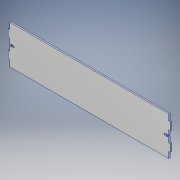
# Autodesk Inventor part: Hopper Leg Brace
Saved by Autodesk Inventor 2018 (Build 220112000, 112)
## iProperties
Created: 2013-10-29
Part Number: Hopper Leg Brace
Material: Aluminum 6061
Document SubType Name: Modeling
Designer: Gabriel Smolnycki
Mass: 474.034 g
Surface Area: 923.52 cm^2
Volume: 175.568 cm^3
Density: 2.7 g/cm^3
Appearance: Aluminum - Flat
Sending System: SolidWorks 2017
Last Author: Gabriel Smolnycki
Last Saved: 2017-09-14
Author: Gabriel Smolnycki
Autodesk Inventor part; units mm, degrees
ref_plane "YZ Plane" through (0, 0, 0) normal (1, 0, 0) x (0, 1, 0)
ref_plane "XZ Plane" through (0, 0, 0) normal (0, 1, 0) x (-1, 0, 0)
ref_plane "Work Plane1" through (0, 0, -4) normal (0, 0, 1) x (1, 0, 0)
sketch "Sketch1" plane through (0, 0, -4) normal (0, 0, 1) x (1, 0, 0)
  line L0 (209, -2.75) -> (209, -1.75)
  line L1 (216, -35) -> (216, -15)
  line L2 (212, -35) -> (216, -35)
  line L3 (209, -1.75) -> (212, -1.75)
  line L4 (-212, -1.75) -> (-209, -1.75)
  line L5 (-212, -51.5) -> (212, -51.5)
  line L6 (-209, -1.75) -> (-209, -2.75)
  line L7 (-212, -35) -> (-212, -51.5)
  line L8 (-216, 15) -> (-212, 15)
  line L9 (-216, -35) -> (-212, -35)
  line L10 (-216, 35) -> (-216, 15)
  line L11 (-209, -2.75) -> (-205, -2.75)
  line L12 (-216, -15) -> (-216, -35)
  line L13 (-212, 35) -> (-216, 35)
  line L14 (-205, -2.75) -> (-205, -1.75)
  line L15 (-212, -15) -> (-216, -15)
  line L16 (-212, 51.5) -> (-212, 35)
  line L17 (-205, -1.75) -> (-200, -1.75)
  line L18 (-212, -1.75) -> (-212, -15)
  line L19 (212, 51.5) -> (-212, 51.5)
  line L20 (-200, -1.75) -> (-200, 1.75)
  line L21 (212, 1.75) -> (209, 1.75)
  line L22 (212, 35) -> (212, 51.5)
  line L23 (-200, 1.75) -> (-205, 1.75)
  line L24 (209, 1.75) -> (209, 2.75)
  line L25 (216, 35) -> (212, 35)
  line L26 (-205, 1.75) -> (-205, 2.75)
  line L27 (209, 2.75) -> (205, 2.75)
  line L28 (-205, 2.75) -> (-209, 2.75)
  line L29 (205, 2.75) -> (205, 1.75)
  line L30 (216, 15) -> (216, 35)
  line L31 (-209, 2.75) -> (-209, 1.75)
  line L32 (205, 1.75) -> (200, 1.75)
  line L33 (212, 15) -> (216, 15)
  line L34 (212, -51.5) -> (212, -35)
  line L35 (-209, 1.75) -> (-212, 1.75)
  line L36 (200, 1.75) -> (200, -1.75)
  line L37 (212, 1.75) -> (212, 15)
  line L38 (-212, 15) -> (-212, 1.75)
  line L39 (200, -1.75) -> (205, -1.75)
  line L40 (205, -1.75) -> (205, -2.75)
  line L41 (212, -15) -> (212, -1.75)
  line L42 (205, -2.75) -> (209, -2.75)
  line L43 (216, -15) -> (212, -15)
  constraints: 88 end point, 29 equal length, 22 horizontal, 22 vertical, 4 collinear
extrude "Extrusion1" add sketch "Sketch1" along normal blind 4.064
body "Solid3"
